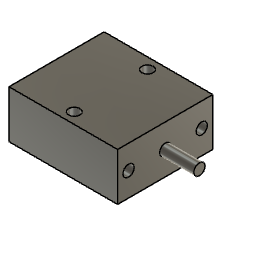
motorholder (Autodesk Fusion 360 design; units mm, degrees)
Autodesk Fusion 360 part; units mm, degrees
note: some values were not read from the file. Set by a fixed rule: which sketch regions a step uses.
sketch "スケッチ1" plane through (0, 0, 0) normal (0, 0, 1) x (1, 0, 0)
  line L0 (0, 0) -> (29, 0)
  line L1 (29, 0) -> (29, 25.4)
  line L2 (29, 25.4) -> (0, 25.4)
  line L3 (0, 25.4) -> (0, 0)
  dimension "d1" = 29
  dimension "d2" = 25.4
  constraint coincident L0.start L3.end
  constraint horizontal L0
  constraint perpendicular L0 L1
  constraint perpendicular L1 L2
  constraint perpendicular L0 L3
  measures "d1" distance of L0.start L0.end
  measures "d2" distance of L0.end L1.end
extrude "押し出し2" add sketch "スケッチ1" along normal blind 12.7 makes body 1
sketch "スケッチ2" plane through (0, 0, 12.7) normal (0, 0, 1) x (-1, 0, 0)
  line L0 (0, -25.4) -> (0, 0)
  line L1 (0, 0) -> (-29, 0)
  line L2 (-29, 0) -> (-29, -25.4)
  line L3 (-29, -25.4) -> (0, -25.4)
  line L4 (-29, -12.7) -> (0, -12.7)
  line L5 (-14.5, -12.7) -> (-14.5, -25.4)
  line L6 (-14.5, 0) -> (-14.5, -12.7)
  line L7 (-14.5, -12.7) -> (-14.5, -22.48)
  circle A0 centre (-14.5, -22.48) radius 1.5
  circle A1 centre (-14.5, -2.92) radius 1.5
  dimension "d10" = 9.78
  dimension "d11" = 3
  constraint midpoint L2 L4.start
  constraint midpoint L0 L4.end
  constraint midpoint L4 L5.start
  constraint midpoint L3 L5.end
  constraint midpoint L1 L6.start
  constraint perpendicular L4 L7
  constraint coincident L7.end A0.centre
  constraint symmetric L4 A0 A1
  measures "d10" distance of L5.start L7.end
  measures "d11" diameter of A0
sketch "スケッチ3" plane through (29, 0, 0) normal (1, 0, 0) x (0, 1, 0)
  line L0 (0, 0) -> (25.4, 0)
  line L1 (25.4, 0) -> (25.4, 12.7)
  line L2 (25.4, 12.7) -> (0, 12.7)
  line L3 (0, 12.7) -> (0, 0)
  line L4 (22.4716, 12.7) -> (22.4716, 0)
  line L5 (2.9158, 12.7) -> (2.9158, 0)
  line L6 (0, 6.35) -> (25.4, 6.35)
  circle A0 centre (2.9158, 6.35) radius 1.5
  circle A1 centre (22.4716, 6.35) radius 1.5
  line L7 (12.7, 12.7) -> (12.7, 0)
  circle A2 centre (12.7, 6.35) radius 1.5
  dimension "d12" = 3
  dimension "d13" = 3
  dimension "d14" = 3
  constraint coincident L2 L4.start
  constraint coincident L0 L4.end
  constraint perpendicular L0 L4
  constraint coincident L2 L5.start
  constraint coincident L0 L5.end
  constraint perpendicular L0 L5
  constraint midpoint L3 L6.start
  constraint midpoint L1 L6.end
  constraint midpoint L5 A0.centre
  constraint midpoint L4 A1.centre
  constraint midpoint L2 L7.start
  constraint midpoint L0 L7.end
  constraint midpoint L7 A2.centre
  measures "d12" diameter of A0
  measures "d13" diameter of A1
  measures "d14" diameter of A2
sketch "スケッチ4" plane through (0, 0, 0) normal (-1, 0, 0) x (0, -1, 0)
  line L0 (-25.4, 0) -> (0, 0)
  line L1 (0, 0) -> (0, 12.7)
  line L2 (0, 12.7) -> (-25.4, 12.7)
  line L3 (-25.4, 12.7) -> (-25.4, 0)
  line L4 (-22.4672, 12.7) -> (-22.4672, 0)
  line L5 (-2.918, 12.7) -> (-2.918, 0)
  line L6 (-25.4, 6.35) -> (0, 6.35)
  circle A0 centre (-22.4672, 6.35) radius 1.5
  circle A1 centre (-2.918, 6.35) radius 1.5
  dimension "d15" = 3
  dimension "d16" = 3
  constraint coincident L2 L4.start
  constraint coincident L0 L4.end
  constraint perpendicular L0 L4
  constraint coincident L2 L5.start
  constraint coincident L0 L5.end
  constraint perpendicular L0 L5
  constraint midpoint L3 L6.start
  constraint midpoint L1 L6.end
  constraint midpoint L4 A0.centre
  constraint midpoint L5 A1.centre
  measures "d15" diameter of A0
  measures "d16" diameter of A1
extrude "押し出し3" cut sketch "スケッチ4" against normal blind 9.144 contours L5 L6 A1 | L5 L6 A1 | L5 L6 A1 | L5 L6 A1 bodies 1
extrude "押し出し4" cut sketch "スケッチ4" against normal blind 9.144 contours L4 L6 A0 | L4 L6 A0 | L4 L6 A0 | L4 L6 A0 bodies 1
extrude "押し出し5" cut sketch "スケッチ2" against normal up to surface (12.7 mm away) contours L6 A1 | L6 A1 bodies 1
extrude "押し出し6" cut sketch "スケッチ2" against normal up to surface (12.7 mm away) contours L5 L7 A0 | L5 L7 A0 bodies 1
extrude "押し出し7" cut sketch "スケッチ3" against normal blind 9.144 contours L5 L6 A0 | L5 L6 A0 | L5 L6 A0 | L5 L6 A0 bodies 1
extrude "押し出し8" cut sketch "スケッチ3" against normal blind 9.144 contours L4 L6 A1 | L4 L6 A1 | L4 L6 A1 | L4 L6 A1 bodies 1
extrude "押し出し9" add sketch "スケッチ3" along normal blind 9.144 contours L6 L7 A2 | L6 L7 A2 | L6 L7 A2 | L6 L7 A2 bodies 1
copy_body "ボディ -> コンポーネント1" bodies 1 removing the originals makes body 2 in component "モーターホルダー1"
extrude "押し出し1" [suppressed]
component "モーターホルダー1" placed x (1, 0, 0) y (0, 1, 0) z (0, 0, 1) at (0, 0, 0)
